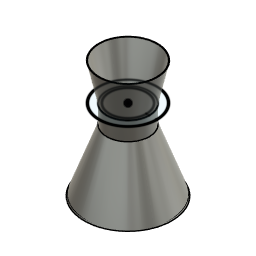
熔岩灯2 (Autodesk Fusion 360 design; units mm, degrees)
Autodesk Fusion 360 part; units mm, degrees
sketch "草图1" plane through (0, 0, 0) normal (0, 1, 0) x (1, 0, 0)
  circle A0 centre (0, 0) radius 46.5
  circle A1 centre (0, 0) radius 47.5
  circle A2 centre (0, 0) radius 33.5
  circle A3 centre (0, 0) radius 34.5
  circle A4 centre (0, 0) radius 45.5
  circle A5 centre (0, 0) radius 30
  circle A6 centre (0, 0) radius 29
  circle A7 centre (0, 0) radius 31
  dimension "d1" = 93
  dimension "d2" = 95
  dimension "d5" = 67
  dimension "d6" = 69
  dimension "d21" = 91
  dimension "d26" = 60
  dimension "d29" = 58
  dimension "d30" = 62
  constraint coincident A0.centre A1.centre
  constraint concentric A0 A2
  constraint concentric A2 A4
  constraint concentric A1 A5
  constraint concentric A2 A6
  constraint concentric A6 A7
  measures "d1" diameter of A0
  measures "d2" diameter of A1
  measures "d5" diameter of A2
  measures "d6" diameter of A3
  measures "d21" diameter of A4
  measures "d26" diameter of A5
  measures "d29" diameter of A6
  measures "d30" diameter of A7
extrude "拉伸8" add sketch "草图1" along normal blind 60 draft 12.3 contours A3
extrude "拉伸9" cut sketch "草图1" along normal blind 60 draft 12.3 contours A2 | A5 | A6 | A7
extrude "拉伸11" add sketch "草图1" against normal blind 30 contours A3
sketch "草图5" plane through (0, -30, 0) normal (0, -1, 0) x (1, 0, 0)
  circle A0 centre (0, 0) radius 33.5
  circle A1 centre (0, 0) radius 34.5
extrude "拉伸13" add sketch "草图5" along normal blind 100 draft 20
extrude "拉伸14" cut sketch "草图5" along normal blind 100 draft 20 contours A0
sketch "草图6" plane through (0, -130, 0) normal (0, -1, 0) x (1, 0, 0)
  circle A0 centre (0, 0) radius 69.897
  circle A1 centre (0, 0) radius 70.897
extrude "拉伸15" add sketch "草图6" against normal blind 2 draft -20 contours A0
